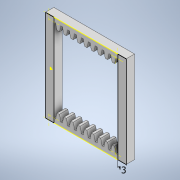
# Autodesk Inventor part: Pinion Rack M 0.9
Saved by Autodesk Inventor 2020.2 (Build 242310000, 310)
## iProperties
Created: 2020-03-13
Part Number: Pinion Rack M 0.9
Material: Generisch
Document SubType Name: Modeling
Designer: JochenAlt
Density: 1 g/cm^3
Appearance: Vorgabe
Author: JochenAlt
Autodesk Inventor part; units mm, degrees
ref_plane "YZ Plane" through (0, 0, 0) normal (1, 0, 0) x (0, 1, 0)
ref_plane "XZ Plane" through (0, 0, 0) normal (0, 1, 0) x (-1, 0, 0)
ref_plane "XY Plane" through (0, 0, 0) normal (0, 0, 1) x (1, 0, 0)
sketch "Skizze1" plane through (0, 0, 0) normal (0, 0, 1) x (1, 0, 0)
  line L0 (0, -22.9152) -> (0, 22.9152) construction
  line L1 (-7.5921, 0) -> (7.5921, 0) construction
  line L2 (-0.4, -12.8) -> (0.4, -12.8)
  arc A0 (-0.4, -12.8) -> (-0.88, -14.868) centre (5.423, -15.2413) ccw
  arc A1 (0.88, -14.868) -> (0.4, -12.8) centre (-5.423, -15.2413) ccw
  line L3 (0.88, -14.868) -> (1.585, -14.868)
  line L4 (-0.88, -14.868) -> (-0.88, -16.368)
  line L5 (-0.88, -16.368) -> (1.585, -16.368)
  line L6 (1.585, -14.868) -> (1.585, -16.368)
  line L7 (-0.4, 12.8) -> (0.4, 12.8)
  arc A2 (-0.88, 14.868) -> (-0.4, 12.8) centre (5.423, 15.2413) ccw
  arc A3 (0.4, 12.8) -> (0.88, 14.868) centre (-5.423, 15.2413) ccw
  line L8 (0.88, 14.868) -> (1.585, 14.868)
  line L9 (-0.88, 14.868) -> (-0.88, 16.368)
  line L10 (-0.88, 16.368) -> (1.585, 16.368)
  line L11 (1.585, 14.868) -> (1.585, 16.368)
  point P0 (0, 0)
  dimension "d0" = 0.8
  dimension "d1" = 6.314
  dimension "d2" = 1.76
  dimension "d3" = 2.068
  dimension "d4" = 0.705
  dimension "d5" = 1.5
  dimension "d11" = 2.465
  dimension "d18" = 25.6
  constraints: 20 end point, 9 symmetric about line, 8 point on circle, 4 centre point, 2 horizontal, 2 perpendicular, 2 point on line, 1 equal radius, 3 other
  measures "d0" distance of L2.start L2.end
  measures "d1" radius of A0
  measures "d2" distance of L3.start L4.start
  measures "d3" distance between parallel lines of L3 L2
  measures "d4" distance of L3.start L3.end
  measures "d5" distance of L3.end L5.end
  measures "d11" distance between parallel lines of L6 L4
  measures "d18" distance of L7.start L2.start
extrude "Extrusion1" add sketch "Skizze1" along normal blind 3
pattern_linear "Rechteckige Anordnung1" count 10 spacing 2.465 along (1, 0, 0)
sketch "Skizze2" plane through (0, 0, 3) normal (0, 0, 1) x (1, 0, 0)
  line L0 (0.88, 16.368) -> (0.88, -16.368)
  line L1 (0.88, -16.368) -> (-2.12, -16.368)
  line L2 (23.77, 16.368) -> (-0.88, 16.368) projected
  line L3 (23.77, 16.368) -> (26.77, 16.368)
  line L4 (26.77, 16.368) -> (26.77, -16.368)
  line L5 (-0.88, -16.368) -> (23.77, -16.368) projected
  line L6 (26.77, -16.368) -> (23.77, -16.368)
  line L7 (23.77, -16.368) -> (23.77, 16.368)
  line L8 (-2.12, -16.368) -> (-2.12, 16.368)
  line L9 (-2.12, 16.368) -> (0.88, 16.368)
  point P0 (0, 0)
  point P1 (23.065, -14.868)
  point P2 (23.065, 14.868)
  point P3 (0.88, 14.868)
  point P4 (0.88, -14.868)
  point P5 (23.77, 14.868)
  point P6 (-0.88, 16.368)
  dimension "d15" = 3
  constraints: 16 end point, 4 perpendicular, 3 point on line, 2 vertical, 1 collinear, 1 horizontal, 1 parallel
  measures "d15" distance of L4.end L5.end
extrude "Extrusion2" cut sketch "Skizze2" against normal up to surface (3 mm away) contours L0 L1 L8 L9 L2
extrude "Extrusion3" add sketch "Skizze2" against normal up to surface (3 mm away) contours L0 L1 L8 L9 L2 | L3 L4 L6 L7
equation "\"d10\" = d11"
